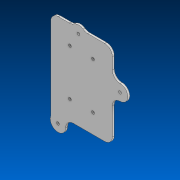
# Autodesk Inventor part: Brain Mount
Saved by Autodesk Inventor 2022 (Build 260153000, 153)
## iProperties
Created: 2022-04-13
Part Number: Brain Mount
Material: Generic
Document SubType Name: Modeling
Designer: score_nygvs6w
Density: 1 g/cm^3
Appearance: Default
Author: score_nygvs6w
Autodesk Inventor part; units mm, degrees
ref_plane "YZ Plane" through (0, 0, 0) normal (1, 0, 0) x (0, 1, 0)
ref_plane "XZ Plane" through (0, 0, 0) normal (0, 1, 0) x (-1, 0, 0)
ref_plane "XY Plane" through (0, 0, 0) normal (0, 0, 1) x (1, 0, 0)
sketch "Sketch1" plane through (0, 0, 0) normal (0, 0, 1) x (1, 0, 0)
  line L0 (19.05, 38.1) -> (-19.05, 38.1) construction
  line L1 (-19.05, 38.1) -> (-19.05, -38.1) construction
  line L2 (-19.05, -38.1) -> (19.05, -38.1) construction
  line L3 (19.05, -38.1) -> (19.05, 38.1) construction
  line L4 (19.05, 38.1) -> (-19.05, -38.1) construction
  line L5 (-19.05, 38.1) -> (19.05, -38.1) construction
  line L6 (-50.8, -69.85) -> (38.1, -69.85)
  line L7 (50.8, -57.15) -> (50.8, 57.15)
  line L8 (38.1, 69.85) -> (-38.1, 69.85)
  line L9 (-50.8, 57.15) -> (-50.8, -69.85)
  line L10 (-50.8, -69.85) -> (50.8, 69.85) construction
  line L11 (50.8, -69.85) -> (-50.8, 69.85) construction
  circle A0 centre (-4.9961, 62.0227) radius 12.7
  circle A1 centre (63.5, 12.7) radius 12.7
  circle A2 centre (-38.7853, -82.55) radius 12.7
  arc A3 (-19.9557, 69.85) -> (-12.4759, 72.2864) centre (-19.9557, 82.55) ccw
  arc A4 (2.4837, 72.2864) -> (9.9635, 69.85) centre (9.9635, 82.55) ccw
  arc A5 (50.8, 38.1) -> (63.5, 25.4) centre (63.5, 38.1) ccw
  arc A6 (63.5, 0) -> (50.8, -12.7) centre (63.5, -12.7) ccw
  arc A7 (-13.3853, -69.85) -> (-26.0853, -82.55) centre (-13.3853, -82.55) ccw
  line L12 (-50.8, -86.6654) -> (-50.8, -69.85)
  arc A8 (38.1, -69.85) -> (50.8, -57.15) centre (38.1, -57.15) ccw
  arc A9 (50.8, 57.15) -> (38.1, 69.85) centre (38.1, 57.15) ccw
  arc A10 (-38.1, 69.85) -> (-50.8, 57.15) centre (-38.1, 57.15) ccw
  point P0 (0, 0)
  point P1 (-38.7853, -69.85)
  point P2 (-50.8, -78.4346)
  dimension "d0" = 38.1
  dimension "d1" = 76.2
  dimension "d2" = 31.75
  dimension "d3" = 31.75
  dimension "d13" = 25.4
  dimension "d20" = 12.7
  constraints: 26 end point, 22 point on circle, 18 tangent, 11 centre point, 11 point on line, 9 equal radius, 7 coincident, 4 midpoint, 4 parallel, 2 horizontal, 2 perpendicular, 1 vertical
  measures "d0" distance of L2.end L1.end
  measures "d1" distance of L1.end L0.end
  measures "d2" distance between parallel lines of L0 L8
  measures "d3" distance between parallel lines of L9 L1
  measures "d13" diameter of A0
  measures "d20" radius of A8
extrude "Extrusion1" add sketch "Sketch1" along normal blind 3.175
hole "Hole1" at (-19.05, 38.1, 0) at (19.05, 38.1, 0) at (19.05, -38.1, 0) at (-19.05, -38.1, 0) at (-38.7853, -82.55, 0) at (63.5, 12.7, 0) at (-4.9961, 62.0227, 0) direction (0, 0, 1) diameter 4.572 end through all
body "Solid1"
